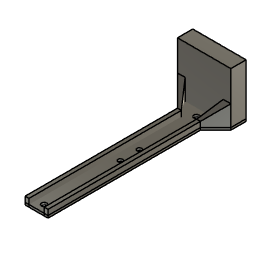
Mini_VESA_Shelf (Autodesk Fusion 360 design; units mm, degrees)
Autodesk Fusion 360 part; units mm, degrees
sketch "Sketch1" plane through (0, 0, 0) normal (0, 0, 1) x (1, 0, 0)
  line L0 (0, 0) -> (30, 0)
  line L1 (30, 0) -> (30, 200)
  line L2 (30, 200) -> (0, 200)
  line L3 (0, 200) -> (0, 0)
  line L4 (5, 200) -> (5, 0)
  line L5 (25, 200) -> (25, 0)
  line L6 (-20, 240) -> (50, 240)
  line L7 (50, 240) -> (50, 220)
  line L8 (50, 220) -> (-20, 220)
  line L9 (-20, 220) -> (-20, 240)
  line L10 (0, 200) -> (-20, 220)
  line L11 (30, 200) -> (50, 220)
  line L12 (25, 200) -> (40, 220)
  line L13 (5, 200) -> (-10, 220)
  line L14 (15, 220) -> (15, 0) construction
  circle A0 centre (15, 210) radius 3.55
  circle A1 centre (15, 10) radius 3.55
  circle A2 centre (15, 110) radius 3.05
  circle A3 centre (15, 135) radius 3.05
  dimension "Bottom_width" = 30
  dimension "Bottom_height" = 200
  dimension "Reinforcement_width" = 5
  dimension "d4" = 5
  dimension "d5" = 70
  dimension "Shelf_height" = 20
  dimension "Transition_section" = 20
  dimension "d8" = 10
  dimension "d9" = 10
  dimension "d10" = 10
  dimension "M8_screw" = 7.1
  dimension "d12" = 7.1
  dimension "VESA200" = 200
  dimension "M6_screw" = 6.1
  dimension "VESA100" = 100
  dimension "d16" = 6.1
  dimension "VESA75" = 75
  constraint horizontal L0
  constraint vertical L1
  constraint horizontal L2
  constraint vertical L3
  constraint coincident L0.start L3.end
  constraint coincident L2 L4.start
  constraint coincident L0 L4.end
  constraint perpendicular L0 L4
  constraint coincident L2 L5.start
  constraint coincident L0 L5.end
  constraint perpendicular L0 L5
  constraint horizontal L6
  constraint vertical L7
  constraint horizontal L8
  constraint vertical L9
  constraint equal L10 L11
  constraint coincident L8 L12.end
  constraint coincident L8 L13.end
  constraint midpoint L8 L14.start
  constraint midpoint L0 L14.end
  constraint coincident L14 A0.centre
  constraint coincident L14 A1.centre
  constraint coincident L14 A2.centre
  constraint coincident L14 A3.centre
  measures "Bottom_width" distance of L0.start L0.end
  measures "Bottom_height" distance of L0.end L1.end
  measures "Reinforcement_width" distance of L3 L4
  measures "d4" distance of L0.end L5.end
  measures "d5" distance of L6.start L6.end L5
  measures "Shelf_height" distance of L6.start L8.end L5
  measures "Transition_section" distance of L2 L8
  measures "d8" distance of L8.end L13.end L5
  measures "d9" distance of L7.end L12.end
  measures "d10" distance of L14.start A0.centre
  measures "M8_screw" diameter of A0
  measures "d12" diameter of A1
  measures "VESA200" distance of A0.centre A1.centre
  measures "M6_screw" diameter of A2
  measures "VESA100" distance of A0.centre A2.centre
  measures "d16" diameter of A3
  measures "VESA75" distance of A0.centre A3.centre
extrude "Extrude Base" add sketch "Sketch1" along normal blind 3 makes body 1
extrude "Extrude Shelf" add sketch "Sketch1" along normal blind 70 separate body contours L6 L7 L8 L9 makes body 2
extrude "Extrude Base Reinforcement" add sketch "Sketch1" along normal blind 10 separate body contours L0 L2 L3 L4 | L0 L1 L2 L5 makes body 3 at (0, 133.3333, 3.3333) makes body 4 at (25, 133.3333, 3.3333)
extrude "Extrude4" add sketch "Sketch1" along normal blind 30 separate body contours L2 L8 L10 L13 | L2 L8 L11 L12 makes body 5 at (-6.6667, 206.6667, 10) makes body 6 at (36.6667, 206.6667, 20)
chamfer "Chamfer1" distance 20 distance2 20 1 edges at (27.5, 200, 30) measured on face at (40, 213.3333, 30) on bodies 6
chamfer "Chamfer2" distance 20 distance2 20 1 edges at (2.5, 200, 30) measured on face at (-10, 213.3333, 30) on bodies 5
equation "d4 = Reinforcement_width"
equation "d8 = Reinforcement_width * 2"
equation "d9 = Reinforcement_width * 2"
equation "d10 = Transition_section / 2"
equation "d12 = M8_screw"
equation "d16 = M6_screw"
